Servo Arm v2 (Autodesk Fusion 360 design; units mm, degrees)
Autodesk Fusion 360 part; units mm, degrees
sketch "Sketch4" plane through (0, 0, 0) normal (0, 0, 1) x (1, 0, 0)
  circle A0 centre (0, 0) radius 3
  circle A1 centre (0, 0) radius 6
  dimension "d9" = 6
  dimension "d10" = 3
  measures "d9" diameter of A0
  measures "d10" distance of A0 A1
extrude "Extrude2" add sketch "Sketch4" along normal blind 3.25
sketch "Sketch5" plane through (0, 0, 3.25) normal (0, 0, 1) x (1, 0, 0)
  circle A0 centre (0, 0) radius 3
  circle A1 centre (0, 0) radius 6
  circle A2 centre (0, 0) radius 1.6
  dimension "d13" = 3.2
  measures "d13" diameter of A2
extrude "Extrude3" add sketch "Sketch5" along normal blind 2.75 contours A0 | A1
sketch "Sketch8" plane through (0, 0, 6) normal (0, 0, 1) x (1, 0, 0)
  circle A0 centre (0, 0) radius 1.6
  circle A1 centre (0, 0) radius 6
  circle A2 centre (0, 0) radius 10
  line L0 (0, -10) -> (0, 10) construction
  line L1 (0, -10) -> (-120, -10)
  line L2 (0, 10) -> (-120, 10)
  circle A3 centre (-120, 0) radius 10
  line L3 (-120, -10) -> (-120, 10) construction
  dimension "d30" = 20
  dimension "d31" = 120
  dimension "d32" = 120
  measures "d30" diameter of A2
  measures "d31" distance of L0.start L1.end
  measures "d32" distance of L0.end L2.end
extrude "Extrude5" add sketch "Sketch8" against normal up to surface (6 mm away) contours A2 | A2 L1 L2 A3 | A3
